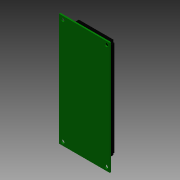
# Autodesk Inventor part: lcd05-16x2
Saved by Autodesk Inventor 2015 (Build 190159000, 159)
## iProperties
Created: 2015-10-31
Part Number: lcd05-16x2
Material: Generic
Document SubType Name: Modeling
Designer: James
Density: 1 g/cm^3
Appearance: Default
Author: James
Autodesk Inventor part; units mm, degrees
ref_plane "YZ Plane" through (0, 0, 0) normal (1, 0, 0) x (0, 1, 0)
ref_plane "XZ Plane" through (0, 0, 0) normal (0, 1, 0) x (-1, 0, 0)
ref_plane "XY Plane" through (0, 0, 0) normal (0, 0, 1) x (1, 0, 0)
sketch "Sketch1" plane through (0, 0, 0) normal (0, 1, 0) x (-1, 0, 0)
  line L0 (-18, 40) -> (-18, -40)
  line L1 (-18, -40) -> (18, -40)
  line L2 (18, -40) -> (18, 40)
  line L3 (18, 40) -> (-18, 40)
  line L4 (-18, 40) -> (18, -40) construction
  line L5 (-18, -40) -> (18, 40) construction
  line L6 (18, 40) -> (-0.55, 40)
  line L7 (18, 40) -> (15.5, 40)
  line L8 (15.5, 40) -> (15.5, 37.5)
  circle A0 centre (15.5, 37.5) radius 1.25
  line L9 (15.5, 37.5) -> (-15.5, 37.5)
  line L10 (-15.5, 37.5) -> (-15.5, -37.5)
  line L11 (-15.5, -37.5) -> (15.5, -37.5)
  circle A1 centre (-15.5, 37.5) radius 1.25
  circle A2 centre (-15.5, -37.5) radius 1.25
  circle A3 centre (15.5, -37.5) radius 1.25
  point P0 (0, 0)
  dimension "d0" = 80
  dimension "d1" = 36
  dimension "d2" = 18.55
  dimension "d25" = 2.5
  dimension "d26" = 2.5
  dimension "d27" = 2.5
  dimension "d28" = 31
  dimension "d29" = 75
  dimension "d30" = 31
  dimension "d31" = 2.5
  dimension "d32" = 2.5
  dimension "d33" = 2.5
  constraints: 24 end point, 4 centre point, 4 coincident, 3 parallel, 3 perpendicular, 2 midpoint, 2 point on line, 1 horizontal, 1 vertical
  measures "d0" distance of L0.start L0.end
  measures "d1" distance of L1.end L0.end
  measures "d2" distance of L2.end L6.end
  measures "d25" distance of L2.end L7.end
  measures "d26" distance of L7.end L8.end
  measures "d27" diameter of A0
  measures "d28" distance of L9.start L9.end
  measures "d29" distance of L9.end L10.end
  measures "d30" distance of L10.end L11.end
  measures "d31" diameter of A1
  measures "d32" diameter of A2
  measures "d33" diameter of A3
extrude "Extrusion1" add sketch "Sketch1" along normal blind 1 contours A3 | A2 L11 L10 | L10 L11 A2 | A1 L10 L9 | L9 L10 A1 | A0 L9 L8 | L8 L9 A0 | L3 L2 L1 L0
sketch "Sketch2" plane through (0, 1, 0) normal (0, 1, 0) x (1, 0, 0)
  line L0 (18, -40) -> (18, 40) projected
  line L1 (18, 40) -> (-18, 40) projected
  line L2 (-18, 40) -> (-18, -40) projected
  line L3 (-18, -40) -> (18, -40) projected
  line L4 (-18, -40) -> (0.55, -40)
  line L5 (-18, -40) -> (18, -40) projected
  line L6 (-11.6, -35.65) -> (-11.6, -33.65)
  line L7 (-11.6, -33.65) -> (-12.6, -33.65)
  line L8 (12.7, -35.65) -> (12.7, -33.65)
  line L9 (12.7, -33.65) -> (13.7, -33.65)
  line L10 (12.7, 35.65) -> (12.7, 33.65)
  line L11 (12.7, 33.65) -> (13.7, 33.65)
  line L12 (-11.6, 35.65) -> (-11.6, 33.65)
  line L13 (-11.6, 33.65) -> (-12.6, 33.65)
  line L14 (-11.6, -35.65) -> (12.7, -35.65)
  line L15 (13.7, -33.65) -> (13.7, 33.65)
  line L16 (12.7, 35.65) -> (-11.6, 35.65)
  line L17 (-12.6, 33.65) -> (-12.6, -33.65)
  point P0 (0, 0)
  dimension "d10" = 2
  dimension "d12" = 2
  dimension "d14" = 2
  dimension "d16" = 2
  constraints: 26 end point, 3 perpendicular, 3 point on line, 1 horizontal, 1 vertical
  measures "d10" distance of L6.start L6.end
  measures "d12" distance of L8.start L8.end
  measures "d14" distance of L10.start L10.end
  measures "d16" distance of L12.start L12.end
extrude "Extrusion2" add sketch "Sketch2" along normal blind 7 contours L6 L7 L17 L13 L12 L16 L10 L11 L15 L9 L8 L14
fillet "Fillet1" radius 0.5 4 edges at (-12.6, 8, 0) (0.55, 8, -35.65) (13.7, 8, 0) (0.55, 8, 35.65)
sketch "Sketch3" plane through (0, 8, 0) normal (0, 1, 0) x (1, 0, 0)
  line L0 (7, -32.25) -> (7, 32.25)
  line L1 (7, 32.25) -> (-7, 32.25)
  line L2 (-7, 32.25) -> (-7, -32.25)
  line L3 (-7, -32.25) -> (7, -32.25)
  line L4 (7, -32.25) -> (-7, 32.25) construction
  line L5 (7, 32.25) -> (-7, -32.25) construction
  point P0 (0, 0)
  dimension "d20" = 64.5
  dimension "d21" = 14
  constraints: 12 end point, 2 midpoint, 2 parallel, 1 perpendicular, 1 vertical
  measures "d20" distance of L0.start L0.end
  measures "d21" distance of L1.end L0.end
extrude "Extrusion3" cut sketch "Sketch3" against normal blind 1
fillet "Fillet2" radius 0.5 4 edges at (7, 7.5, -32.25) (7, 7.5, 32.25) (-7, 7.5, 32.25) (-7, 7.5, -32.25)
sketch "Sketch4" plane through (0, 1, 0) normal (0, 1, 0) x (1, 0, 0)
  line L0 (-18, 40) -> (-18, -40)
  line L1 (-18, -40) -> (18, -40)
  line L2 (18, -40) -> (18, 40)
  line L3 (18, 40) -> (-18, 40)
  line L4 (-18, 40) -> (18, -40) construction
  line L5 (-18, -40) -> (18, 40) construction
  line L6 (18, 40) -> (-0.55, 40)
  line L7 (18, 40) -> (15.5, 40)
  line L8 (15.5, 40) -> (15.5, 37.5)
  circle A0 centre (15.5, 37.5) radius 1.25
  line L9 (15.5, 37.5) -> (-15.5, 37.5)
  line L10 (-15.5, 37.5) -> (-15.5, -37.5)
  line L11 (-15.5, -37.5) -> (15.5, -37.5)
  circle A1 centre (-15.5, 37.5) radius 1.25
  circle A2 centre (-15.5, -37.5) radius 1.25
  circle A3 centre (15.5, -37.5) radius 1.25
  point P0 (0, 0)
  point P1 (0, 0)
  dimension "d34" = 80
  dimension "d35" = 36
  dimension "d36" = 18.55
  dimension "d37" = 2.5
  dimension "d38" = 2.5
  dimension "d39" = 2.5
  dimension "d40" = 31
  dimension "d41" = 75
  dimension "d42" = 31
  dimension "d43" = 2.5
  dimension "d44" = 2.5
  dimension "d45" = 2.5
  constraints: 24 end point, 4 centre point, 4 coincident, 3 parallel, 3 perpendicular, 2 midpoint, 2 point on line, 1 horizontal, 1 vertical
  measures "d34" distance of L3.end L5.start
  measures "d35" distance of L2.start L5.start
  measures "d36" distance of L6.start L6.end
  measures "d37" distance of L6.start L7.end
  measures "d38" distance of L7.end L8.end
  measures "d39" diameter of A0
  measures "d40" distance of L9.start L9.end
  measures "d41" distance of L9.end L11.start
  measures "d42" distance of L11.start L11.end
  measures "d43" diameter of A1
  measures "d44" diameter of A2
  measures "d45" diameter of A3
extrude "Extrusion4" cut sketch "Sketch4" against normal blind 1 contours A3 | A2 L11 L10 | L10 L11 A2 | A1 L10 L9 | L9 L10 A1 | A0 L9 L8 | L8 L9 A0
body "Solid1"
